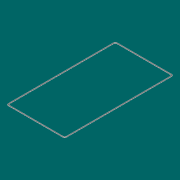
# Autodesk Inventor part: topORing
Saved by Autodesk Inventor 2016 (Build 200138000, 138)
## iProperties
Created: 2015-10-27
Part Number: topORing
Material: Rubber
Document SubType Name: Modeling
Designer: Sawaiz
Density: 0.93 g/cm^3
Appearance: Rubber - Black
Author: Sawaiz
Autodesk Inventor part; units mm, degrees
ref_plane "YZ Plane" through (0, 0, 0) normal (1, 0, 0) x (0, 1, 0)
ref_plane "XZ Plane" through (0, 0, 0) normal (0, 1, 0) x (-1, 0, 0)
ref_plane "XY Plane" through (0, 0, 0) normal (0, 0, 1) x (1, 0, 0)
sketch "Sketch1" plane through (0, 0, 0) normal (0, 0, 1) x (1, 0, 0)
  line L0 (111.125, -60.325) -> (-111.125, -60.325)
  line L1 (-111.125, -60.325) -> (-111.125, 60.325)
  line L2 (-111.125, 60.325) -> (111.125, 60.325)
  line L3 (111.125, 60.325) -> (111.125, -60.325)
  line L4 (111.125, -60.325) -> (-111.125, 60.325) construction
  line L5 (-111.125, -60.325) -> (111.125, 60.325) construction
  line L6 (-109.5375, 54.3179) -> (-109.5375, -54.3179)
  line L7 (-105.1179, -58.7375) -> (105.1179, -58.7375)
  line L8 (109.5375, -54.3179) -> (109.5375, 54.3179)
  line L9 (105.1179, 58.7375) -> (-105.1179, 58.7375)
  line L10 (-107.3277, -54.3179) -> (-107.3277, 54.3179)
  line L11 (-105.1179, 56.5277) -> (105.1179, 56.5277)
  line L12 (107.3277, 54.3179) -> (107.3277, -54.3179)
  line L13 (105.1179, -56.5277) -> (-105.1179, -56.5277)
  arc A0 (-107.3277, -54.3179) -> (-105.1179, -56.5277) centre (-105.1179, -54.3179) ccw
  arc A1 (105.1179, -56.5277) -> (107.3277, -54.3179) centre (105.1179, -54.3179) ccw
  arc A2 (107.3277, 54.3179) -> (105.1179, 56.5277) centre (105.1179, 54.3179) ccw
  arc A3 (-105.1179, 56.5277) -> (-107.3277, 54.3179) centre (-105.1179, 54.3179) ccw
  arc A4 (-109.5375, -54.3179) -> (-105.1179, -58.7375) centre (-105.1179, -54.3179) ccw
  arc A5 (105.1179, -58.7375) -> (109.5375, -54.3179) centre (105.1179, -54.3179) ccw
  arc A6 (109.5375, 54.3179) -> (105.1179, 58.7375) centre (105.1179, 54.3179) ccw
  arc A7 (-105.1179, 58.7375) -> (-109.5375, 54.3179) centre (-105.1179, 54.3179) ccw
  point P0 (0, 0)
  dimension "d0" = 222.25
  dimension "d1" = 120.65
  dimension "d2" = 1.5875
  dimension "d3" = 2.2098
  dimension "d4" = 2.2098
  dimension "d5" = 4.4196
  constraints: 28 end point, 16 point on circle, 16 tangent, 8 centre point, 6 equal radius, 6 parallel, 3 perpendicular, 2 midpoint, 1 horizontal, 6 other
  measures "d0" distance of L1.end L2.end
  measures "d1" distance of L0.end L1.end
  measures "d2" distance between parallel lines of L1 L6
  measures "d3" distance between parallel lines of L6 L10
  measures "d4" radius of A0
  measures "d5" radius of A4
extrude "Extrusion1" add sketch "Sketch1" along normal blind 1.1684 contours A7 L9 A6 L8 A5 L7 A4 L6
fillet "Fillet1" radius 0.5 32 edges at (-106.6805, 55.8805, 1.1684) (0, 56.5277, 1.1684) (106.6805, 55.8805, 1.1684) (107.3277, 0, 1.1684) (106.6805, -55.8805, 1.1684) (0, -56.5277, 1.1684) (-106.6805, -55.8805, 1.1684) (-107.3277, 0, 1.1684) (-106.6805, 55.8805, 0) (-107.3277, 0, 0) (-106.6805, -55.8805, 0) (0, -56.5277, 0) (106.6805, -55.8805, 0) (107.3277, 0, 0) (106.6805, 55.8805, 0) (0, 56.5277, 0) (-109.5375, 0, 1.1684) (-108.243, -57.443, 1.1684) (0, -58.7375, 1.1684) (108.243, -57.443, 1.1684) (109.5375, 0, 1.1684) (108.243, 57.443, 1.1684) (0, 58.7375, 1.1684) (-108.243, 57.443, 1.1684) (-109.5375, 0, 0) (-108.243, 57.443, 0) (0, 58.7375, 0) (108.243, 57.443, 0) (109.5375, 0, 0) (108.243, -57.443, 0) (0, -58.7375, 0) (-108.243, -57.443, 0)
equation "\"d0\" = depth + 2 * frameAcrylicThickness"
equation "\"d1\" = width + 2 * frameAcrylicThickness"
equation "\"frameAcrylicThickness\" = 9.525"
equation "\"internalAcrylicThickness\" = 6.35"
equation "\"aerogelWidth\" = 101.6"
equation "\"aerogelHeight\" = 101.6"
equation "\"height\" = 101.6"
equation "\"width\" = 101.6"
equation "\"depth\" = 203.2"
equation "\"mirrorAngle\" = 5deg"
equation "\"detectorWidth\" = 52"
equation "\"detectorHeight\" = 52"
equation "\"mirrorThickness\" = 3.175"
equation "\"fresnelThickness\" = 0.1"
equation "\"focalLength\" = 76.2"
equation "\"ior\" = 1.49"
equation "\"centerThickness\" = 1.524"
equation "\"fresnelAngle\" = 90deg"
equation "\"fresnelEffectiveDiameter\" = 76.2"
equation "\"oRingWidth\" = 1.5875"
equation "\"sensorHolderDepth\" = 19.05"
body "Solid1"
